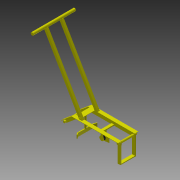
# Autodesk Inventor part: frame
Saved by Autodesk Inventor 2015 (Build 190159000, 159)
## iProperties
Created: 2015-09-11
Part Number: frame
Material: Generic
Document SubType Name: Modeling
Designer: Okorie Ifeanyichukwu
Density: 1 g/cm^3
Appearance: Smooth - Yellow
Author: Okorie Ifeanyichukwu
Autodesk Inventor part; units mm, degrees
sketch "Sketch1" plane through (0, 0, 0) normal (0, 0, 1) x (1, 0, 0)
  line L0 (218.0196, 0) -> (-481.9804, 0)
  line L1 (-481.9804, 0) -> (-635.1893, -128.5575)
  point P0 (0, 0)
  dimension "d0" = 700
  dimension "d1" = 200
  dimension "d2" = 140
  constraints: 4 end point, 1 horizontal
  measures "d0" distance of L0.start L0.end
  measures "d1" distance of L0.end L1.end
  measures "d2" angle of L1 L0
sketch "Sketch2" plane through (0, 0, 0) normal (1, 0, 0) x (0, 1, 0)
  line L0 (26.8704, 39.9961) -> (22.8704, 39.9961)
  line L1 (22.8704, 39.9961) -> (22.8704, -10.661)
  line L2 (26.8704, -10.8039) -> (26.8704, 39.9961)
  line L3 (22.8704, -10.661) -> (-25.9296, -10.661)
  line L4 (-25.9296, -10.661) -> (-25.9296, -14.661)
  line L5 (-25.9296, -14.661) -> (26.8704, -14.661)
  line L6 (26.8704, -14.661) -> (26.8704, -10.661)
  point P0 (0, 0)
  dimension "d3" = 4
  dimension "d4" = 4
  constraints: 14 end point, 3 parallel, 2 horizontal, 2 perpendicular, 1 point on line
  measures "d3" distance between parallel lines of L1 L2
  measures "d4" distance between parallel lines of L5 L3
sweep "Sweep1" add profiles "Sketch2" path "Sketch1"
sketch "Sketch3" plane through (218.0196, -25.9296, -14.661) normal (0, 0, -1) x (-1, 0, 0)
  line L0 (610.6044, 52.8) -> (690.5624, 52.8)
  line L1 (690.5624, 52.8) -> (690.5624, 48.8)
  line L2 (690.5624, 48.8) -> (610.6044, 48.8)
  line L3 (610.6044, 48.8) -> (610.6044, 52.8)
  line L4 (690.5624, 0) -> (690.5624, 66.6309) construction
  line L5 (0, 52.8) -> (709.78, 52.8) projected
  point P0 (218.0196, 25.9296)
  point P1 (690.5624, 50.8)
  point P2 (650.5834, 52.8)
  dimension "d9" = 4
  constraints: 10 end point, 2 midpoint, 2 parallel, 2 point on line, 1 horizontal, 1 perpendicular, 1 vertical
  measures "d9" distance of L2.end L0.start
extrude "Extrusion1" add sketch "Sketch3" along normal blind 200
ref_plane "Work Plane1" through (218.0196, -25.9296, -114.661) normal (0, 0, -1) x (-1, 0, 0)
mirror "Mirror1" about plane through (218.0196, -25.9296, -114.661) normal (0, 0, -1) of "Sweep1"
sketch "Sketch5" plane through (218.0196, 26.8704, 39.9961) normal (0, 1, 0) x (1, 0, 0)
  line L0 (-613.1384, 54.6571) -> (-567.9618, 54.6571)
  line L1 (-567.9618, 54.6571) -> (-567.9618, 19.6801)
  line L2 (-567.9618, 19.6801) -> (-613.1384, 19.6801)
  line L3 (-613.1384, 19.6801) -> (-613.1384, 54.6571)
  point P0 (-218.0196, 39.9961)
  point P1 (-590.5501, 54.6571)
  constraints: 8 end point, 2 parallel, 1 horizontal, 1 midpoint, 1 perpendicular
sketch "Sketch6" plane through (218.0196, -25.9296, -10.661) normal (0, 0, 1) x (1, 0, 0)
  line L0 (0, 52.8) -> (-610.6044, 52.8) projected
  line L1 (-583.5598, 52.8) -> (-1133.5598, 1005.4279)
  line L2 (0, 52.8) -> (-709.78, 52.8) projected
  point P0 (-218.0196, 25.9296)
  point P1 (-354.89, 52.8)
  dimension "d13" = 60
  dimension "d14" = 1100
  constraints: 3 point on line, 2 end point, 1 midpoint
  measures "d13" angle of L1 L2
  measures "d14" distance of L1.start L1.end
sweep "Sweep2" add profiles "Sketch5" path "Sketch6" path curves L1
mirror "Mirror2" about plane through (218.0196, -25.9296, -114.661) normal (0, 0, -1) of "Sweep2"
sketch "Sketch8" plane through (218.0196, -25.9296, -214.661) normal (0, 0, 1) x (1, 0, 0)
  circle A0 centre (-19.5949, 25.9296) radius 15.8445
  point P0 (-218.0196, 25.9296)
  constraints: 1 centre point
extrude "Extrusion2" add sketch "Sketch8" along normal up to next
sketch "Sketch9" plane through (218.0196, -25.9296, -14.661) normal (0, 0, -1) x (-1, 0, 0)
  circle A0 centre (837.0643, -91.8904) radius 16.0278
  point P0 (218.0196, 25.9296)
  constraints: 1 centre point
extrude "Extrusion3" add sketch "Sketch9" along normal up to next
sketch "Sketch10" plane through (218.0196, -25.9296, -14.661) normal (0, 0, -1) x (-1, 0, 0)
  line L0 (304.1285, 17.4779) -> (304.1285, -78.016) construction
  line L1 (289.2739, 17.4779) -> (289.2739, -78.016)
  line L2 (318.9831, -78.016) -> (318.9831, 17.4779)
  arc A0 (318.9831, 17.4779) -> (289.2739, 17.4779) centre (304.1285, 17.4779) ccw
  arc A1 (289.2739, -78.016) -> (318.9831, -78.016) centre (304.1285, -78.016) ccw
  point P0 (218.0196, 25.9296)
  point P1 (304.1285, -30.2691)
  constraints: 8 end point, 4 point on circle, 4 tangent, 2 centre point, 1 midpoint, 1 parallel, 1 vertical
extrude "Extrusion4" add sketch "Sketch10" along normal blind 10
sketch "Sketch11" plane through (-100.9634, -103.9455, -14.661) normal (-1, 0, 0) x (0, 0, 1)
  line L0 (-10, 95.4938) -> (-10, 0) construction
  line L1 (-43.2722, 25.0503) -> (-20.6673, 25.0503)
  line L2 (-20.6673, 25.0503) -> (-19.5312, 33.0034)
  line L3 (-19.5312, 33.0034) -> (-13.965, 33.0034)
  line L4 (-13.965, 33.0034) -> (-13.965, 12.224)
  line L5 (-13.965, 12.224) -> (-50.3413, 12.224)
  line L6 (-50.3413, 12.224) -> (-50.3413, 33.0034)
  line L7 (-44.7059, 33.0034) -> (-43.2722, 25.0503)
  line L8 (-44.7059, 33.0034) -> (-50.3413, 33.0034)
  line L9 (-10, 0) -> (-79.3915, 0)
  point P0 (14.661, 103.9455)
  constraints: 18 end point, 3 horizontal, 3 perpendicular, 1 parallel
revolve "Revolution1" add sketch "Sketch11" angle 360 about axis through (-100.9634, -103.9455, -24.661) along (0, 0, -1)
sketch "Sketch12" plane through (-100.9634, -103.9455, -28.626) normal (0, 0, 1) x (1, 0, 0)
  circle A0 centre (0, 0) radius 12.224 projected
  point P0 (100.9634, 103.9455)
extrude "Extrusion5" add sketch "Sketch12" along normal blind 5.2375
sketch "Sketch13" plane through (-472.5428, 22.8704, -14.661) normal (0, -1, 0) x (1, 0, 0)
  line L0 (79.958, 0) -> (79.958, -200) construction
  line L1 (79.958, -100) -> (-28.5864, -100) construction
  circle A0 centre (37.9228, -100) radius 12.7611
  point P0 (472.5428, 14.661)
  constraints: 2 end point, 1 centre point, 1 horizontal, 1 midpoint, 1 point on line
extrude "Extrusion6" add sketch "Sketch13" along normal blind 200
ref_plane "Work Plane2" through (-432.5638, 26.8704, -214.661) normal (-1, 0, 0) x (0, 0, 1)
sketch "Sketch14" plane through (-432.5638, 26.8704, -214.661) normal (-1, 0, 0) x (0, 0, 1)
  line L0 (87.2389, -204) -> (112.7611, -204) projected
  line L1 (87.2389, -204) -> (112.7611, -204) projected
  line L2 (112.7611, -4) -> (87.2389, -4) projected
  line L3 (87.2389, -204) -> (-17.7965, -204)
  line L4 (112.7611, -204) -> (219.716, -204)
  line L5 (-17.7965, -255.893) -> (219.716, -255.893)
  line L6 (-17.7965, -255.893) -> (-17.7965, -204)
  line L7 (219.716, -204) -> (219.716, -255.893)
  point P0 (214.661, -26.8704)
  constraints: 10 end point, 2 horizontal, 1 perpendicular, 1 point on line, 1 vertical
extrude "Extrusion7" add sketch "Sketch14" along normal mid plane 11.5875
ref_plane "Work Plane3" through (-438.3575, -203.0761, -232.4575) normal (0, 1, 0) x (1, 0, 0)
sketch "Sketch15" plane through (-438.3575, -203.0761, -232.4575) normal (0, 1, 0) x (1, 0, 0)
  line L0 (0, 0) -> (16.5795, 45.4136)
  line L1 (16.5795, 45.4136) -> (26.8042, 41.6808)
  line L2 (26.8042, 41.6808) -> (11.5875, 0)
  line L3 (11.5875, 0) -> (11.5875, -237.5125)
  line L4 (11.5875, -127.8575) -> (11.5875, -237.5125) projected
  line L5 (11.5875, -237.5125) -> (30.8538, -264.434)
  line L6 (30.8538, -264.434) -> (22.3558, -270.5155)
  line L7 (22.3558, -270.5155) -> (0, -237.5125)
  line L8 (0, -237.5125) -> (0, 0)
  line L9 (0, -105.595) -> (0, 0) projected
  point P0 (438.3575, -232.4575)
  constraints: 16 end point, 3 perpendicular, 2 collinear, 2 point on line
extrude "Extrusion8" add sketch "Sketch15" along normal mid plane 51.275
sketch "Sketch16" plane through (218.0196, -25.9296, -14.661) normal (0, 0, -1) x (-1, 0, 0)
  line L0 (0, 0) -> (690.5624, 0) projected
  line L1 (313.8718, 0) -> (352.9486, 0)
  line L2 (352.9486, 0) -> (352.9486, 15.0768)
  line L3 (352.9486, 15.0768) -> (313.8718, 15.0768)
  line L4 (313.8718, 15.0768) -> (313.8718, 0)
  point P0 (218.0196, 25.9296)
  constraints: 8 end point, 2 parallel, 1 horizontal, 1 perpendicular, 1 point on line
extrude "Extrusion9" add sketch "Sketch16" along normal up to surface (200 mm away)
sketch "Sketch17" plane through (-472.5428, -25.9296, -10.661) normal (0, -1, 0) x (1, 0, 0)
  line L0 (342.3885, -71.7416) -> (372.8501, -71.7416)
  line L1 (372.8501, -71.7416) -> (372.8501, -94.1702)
  line L2 (372.8501, -94.1702) -> (342.3885, -94.1702)
  line L3 (342.3885, -94.1702) -> (342.3885, -71.7416)
  point P0 (472.5428, 10.661)
  constraints: 8 end point, 2 parallel, 1 horizontal, 1 perpendicular
extrude "Extrusion10" add sketch "Sketch17" along normal blind 70.325
sketch "Sketch18" plane through (-472.5428, -96.2546, -10.661) normal (0, -1, 0) x (1, 0, 0)
  line L0 (333.8039, -108.0225) -> (333.8039, -64.8347)
  line L1 (333.8039, -64.8347) -> (427.428, -79.12)
  line L2 (427.428, -79.12) -> (333.8039, -108.0225)
  point P0 (472.5428, 10.661)
  constraints: 6 end point, 1 vertical
extrude "Extrusion11" add sketch "Sketch18" along normal blind 70.325
sketch "Sketch19" plane through (218.0196, -25.9296, -10.661) normal (0, 0, 1) x (1, 0, 0)
  line L0 (-44.7025, 41.7741) -> (0, 41.7741)
  line L1 (0, 41.7741) -> (0, -255.8937)
  line L2 (0, -255.8937) -> (-44.7025, -255.8937)
  line L3 (-44.7025, -255.8937) -> (-44.7025, 41.7741)
  point P0 (-218.0196, 25.9296)
  constraints: 8 end point, 2 parallel, 1 horizontal, 1 perpendicular
extrude "Extrusion12" add sketch "Sketch19" along normal blind 13.175
ref_plane "Work Plane4" through (218.0196, -25.9296, -114.661) normal (0, 0, -1) x (-1, 0, 0)
mirror "Mirror3" about plane through (218.0196, -25.9296, -114.661) normal (0, 0, -1) of "Extrusion12"
sketch "Sketch20" plane through (173.3171, -281.8233, -218.661) normal (0, 0, 1) x (1, 0, 0)
  line L0 (44.7025, 0) -> (0, 0)
  line L1 (0, 0) -> (0, 12.6685)
  line L2 (0, 12.6685) -> (44.7025, 12.6685)
  line L3 (44.7025, 12.6685) -> (44.7025, 0)
  point P0 (-173.3171, 281.8233)
  constraints: 8 end point, 2 parallel, 1 horizontal, 1 perpendicular
extrude "Extrusion13" add sketch "Sketch20" along normal up to next
sketch "Sketch21" plane through (218.0196, -25.9296, 2.514) normal (0, 0, 1) x (1, 0, 0)
  circle A0 centre (-19.5949, 25.9296) radius 15.8445 projected
  circle A1 centre (-837.0643, -91.8904) radius 16.0278 projected
  point P0 (-218.0196, 25.9296)
extrude "Extrusion14" add sketch "Sketch21" along normal blind 24.2875
mirror "Mirror4" about plane through (218.0196, -25.9296, -114.661) normal (0, 0, -1) of "Extrusion14"
ref_plane "Work Plane5" through (218.0196, -25.9296, -114.661) normal (0, 0, 1) x (1, 0, 0)
sketch "Sketch22" plane through (218.0196, -25.9296, -114.661) normal (0, 0, 1) x (1, 0, 0)
  circle A0 centre (-1140.2348, 1008.9697) radius 21.2143
  point P0 (-218.0196, 25.9296)
  constraints: 1 centre point
extrude "Extrusion15" add sketch "Sketch22" along normal mid plane 646.5875
sketch "Sketch23" plane through (-395.1188, 26.8704, 20.316) normal (0, 0, 1) x (1, 0, 0)
  circle A0 centre (14.5698, 18.9714) radius 9.5199
  point P0 (395.1188, -26.8704)
  constraints: 1 centre point
extrude "Extrusion16" add sketch "Sketch23" along normal blind 10
mirror "Mirror5" about plane through (218.0196, -25.9296, -114.661) normal (0, 0, -1) of "Extrusion16"
equation "\"d4\" = d3"
body "Solid1"
